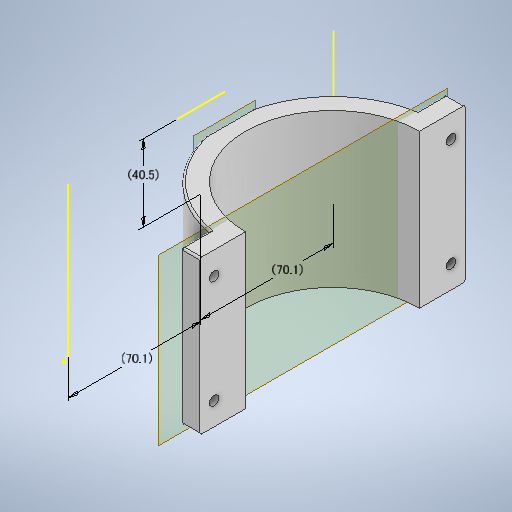
# Autodesk Inventor part: bearing
Saved by Autodesk Inventor 2025.2 (Build 292293000, 293)
## iProperties
Created: 2024-12-14
Part Number: bearing
Material: 一般
Document SubType Name: Modeling
Designer: mahhy
Density: 1 g/cm^3
Appearance: 既定
Author: mahhy
## iProperties of the stored document motor_mount2_3D プリント.ipt
Created: 2024-12-18
Part Number: motor_mount2_3D プリント
Material: 一般
Document SubType Name: Modeling
Designer: mahhy
Density: 1 g/cm^3
Appearance: 既定
Author: mahhy
Autodesk Inventor part; units mm, degrees
ref_plane "YZ Plane" through (0, 0, 0) normal (1, 0, 0) x (0, 1, 0)
ref_plane "XZ Plane" through (0, 0, 0) normal (0, 1, 0) x (-1, 0, 0)
ref_plane "XY Plane" through (0, 0, 0) normal (0, 0, 1) x (1, 0, 0)
sketch "スケッチ1" plane through (0, 0, 0) normal (0, 1, 0) x (-1, 0, 0)
  line L0 (0, 0) -> (70, 0)
  line L1 (70, 0) -> (70, -170)
  line L2 (70, -170) -> (0, -170)
  line L3 (0, -170) -> (0, 0)
  arc A0 (0, -118.5907) -> (0, -26.5907) centre (0, -72.5907) ccw
  arc A1 (0, -128.5907) -> (0, -16.5907) centre (0, -72.5907) ccw
  line L4 (10, -17.4908) -> (0, -17.4908)
  line L5 (0, -17.4908) -> (0, -2.4908)
  line L6 (0, -2.4908) -> (10, -2.4908)
  line L7 (10, -2.4908) -> (10, -17.4908)
  line L8 (10, -127.6907) -> (0, -127.6907)
  line L9 (0, -127.6907) -> (0, -142.6907)
  line L10 (0, -142.6907) -> (10, -142.6907)
  line L11 (10, -142.6907) -> (10, -127.6907)
  line L12 (54.5871, -60.0907) -> (54.5871, -85.0907)
  point P0 (0, -17.4908)
  dimension "d0" = 70
  dimension "d1" = 170
  dimension "d2" = 46
  dimension "d3" = 56
  dimension "d4" = 10
  dimension "d5" = 10
  dimension "d6" = 15
  dimension "d7" = 15
  dimension "d8" = 25
  constraints: 24 end point, 8 point on circle, 5 parallel, 3 horizontal, 3 perpendicular, 2 centre point, 2 vertical, 1 coincident, 10 other
  measures "d0" distance of L1.end L2.end
  measures "d1" distance of L0.end L1.end
  measures "d2" radius of A0
  measures "d3" radius of A1
  measures "d6" distance of L6.end L4.start
  measures "d7" distance of L10.end L8.start
  measures "d8" distance of L12.start L12.end
extrude "押し出し1" add sketch "スケッチ1" along normal blind 81 contours L6 L7 A1 L3 | A1 L4 L3 | L4 A1 L12 L8 L3 A0 | L3 A1 L11 L10 | L3 L8 A1
ref_plane "作業平面1" through (-54.5871, 0, -85.0907) normal (-1, 0, 0) x (0, 0, 1)
sketch "スケッチ2" plane through (-54.5871, 0, -85.0907) normal (-1, 0, 0) x (0, 0, 1)
  line L0 (-33.5, 81) -> (58.5, 81) projected
  line L1 (25, 0) -> (25, 81) projected
  circle A0 centre (12.5, 40.5) radius 12.5
  line L2 (0, 0) -> (0, 81) projected
  line L3 (0, 0) -> (25, 0) projected
  line L4 (-57.5999, 0) -> (-57.5999, 81) projected
  line L5 (82.5999, 0) -> (82.5999, 81) projected
  point P0 (85.0907, 0)
  point P1 (12.5, 0)
  point P2 (-57.5999, 40.5)
  point P3 (82.5999, 40.5)
  dimension "d12" = 25
  dimension "d40" = 70.0999
  dimension "d41" = 70.0999
  constraints: 3 midpoint, 1 centre point, 1 coincident
  measures "d12" diameter of A0
  measures "d40" distance of point (-57.6, 40.5) point (12.5, 40.5)
  measures "d41" distance of point (82.6, 40.5) point (12.5, 40.5)
extrude "押し出し2" add sketch "スケッチ2" along normal blind 5 contours A0
ref_plane "作業平面2" through (-59.5871, 40.5, -72.5907) normal (-1, 0, 0) x (0, 0, 1)
ref_plane "作業平面3" through (-10, 0, -142.6907) normal (-1, 0, 0) x (0, 0, 1)
sketch "スケッチ4" plane through (-10, 0, -142.6907) normal (-1, 0, 0) x (0, 0, 1)
  line L0 (0, 81) -> (15, 81) projected
  line L1 (0, 0) -> (15, 0) projected
  line L2 (125.1998, 0) -> (140.1998, 0) projected
  line L3 (125.1998, 81) -> (140.1998, 81) projected
  point P0 (142.6907, 0)
  point P1 (7.5, 69)
  point P2 (7.5, 12)
  point P3 (132.6998, 12)
  point P4 (132.6998, 69)
  point P5 (7.5, 81)
  point P6 (7.5, 0)
  point P7 (132.6998, 0)
  point P8 (132.6998, 81)
  dimension "d20" = 0
  dimension "d21" = 12
  dimension "d22" = 0
  dimension "d23" = 12
  dimension "d24" = 0
  dimension "d25" = 12
  dimension "d26" = 0
  dimension "d27" = 12
  constraints: 4 midpoint
  measures "d20" horizontal distance of point (7.5, 81) point (7.5, 69)
  measures "d21" distance from line of L0 point (7.5, 69)
  measures "d22" horizontal distance of point (7.5, 0) point (7.5, 12)
  measures "d23" distance from line of L1 point (7.5, 12)
  measures "d24" horizontal distance of point (132.7, 0) point (132.7, 12)
  measures "d25" distance from line of L2 point (132.7, 12)
  measures "d26" horizontal distance of point (132.7, 81) point (132.7, 69)
  measures "d27" distance from line of L3 point (132.7, 69)
hole "穴1" at (-10, 69, -135.1907) at (-10, 12, -135.1907) at (-10, 12, -9.9908) at (-10, 69, -9.9908) direction (1, 0, 0) diameter 5 end through all
fillet "フィレット1" radius 1 16 edges at (-10, 40.5, -2.4908) (-5, 81, -2.4908) (-10, 81, -9.9908) (-38.6854, 81, -32.1008) (-38.6854, 81, -113.0807) (-10, 81, -135.1907) (-5, 81, -142.6907) (-10, 0, -9.9908) (-38.6854, 0, -32.1008) (-5, 0, -2.4908) (-38.6854, 0, -113.0807) (-54.5871, 0, -72.5907) (-10, 0, -135.1907) (-5, 0, -142.6907) (-10, 40.5, -142.6907) (-54.5871, 81, -72.5907)
sketch "スケッチ8" plane through (-59.5871, 40.5, -72.5907) normal (-1, 0, 0) x (0, 0, 1)
  circle A0 centre (0, 0) radius 8.5
  point P0 (72.5907, -40.5)
  dimension "d46" = 17
  constraints: 1 centre point
  measures "d46" diameter of A0
extrude "押し出し4" add sketch "スケッチ8" along normal blind 10
sketch "スケッチ9" plane through (-69.5871, 40.5, -72.5907) normal (-1, 0, 0) x (0, 0, 1)
  circle A0 centre (0, 0) radius 8.5 projected
  line L0 (-70.0999, 39.5) -> (-70.0999, -39.5) projected
  line L1 (12.3865, 40.5) -> (-12.3865, 40.5) projected
  line L2 (70.0999, -39.5) -> (70.0999, 39.5) projected
  point P0 (72.5907, -40.5)
  dimension "d49" = 70.0999
  dimension "d50" = 40.5
  dimension "d51" = 70.0999
  constraints: 1 coincident
  measures "d49" distance from line of L0 point (0, 0)
  measures "d50" distance from line of L1 point (0, 0)
  measures "d51" distance from line of L2 A0.centre
